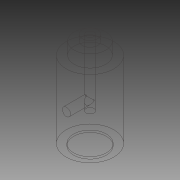
# Autodesk Inventor part: ToolHolderSlug Body
Saved by Autodesk Inventor 2012 SP1 (Build 160190100, 190)
## iProperties
Created: 2010-02-09
Part Number: ToolHolderSlug Body
Document SubType Name: Modeling
Designer: rconnaug
Density: 2.71 g/cm^3
Material: Aluminum-6061
Mass: 6.06549 g
Surface Area: 11.541 cm^2
Volume: 2.23819 cm^3
Author: rconnaug
Autodesk Inventor part; units mm, degrees
ref_plane "YZ Plane" through (0, 0, 0) normal (1, 0, 0) x (0, 1, 0)
ref_plane "XZ Plane" through (0, 0, 0) normal (0, 1, 0) x (-1, 0, 0)
sketch "Sketch1" plane through (0, 0, 0) normal (0, 0, 1) x (1, 0, 0)
  line L0 (0, -4.814) -> (0, 28.884) construction
  line L1 (0.9906, 24.07) -> (1.9304, 24.07)
  line L2 (1.9304, 24.07) -> (1.9304, 22.606)
  line L3 (1.9304, 22.606) -> (3.9497, 22.606)
  line L4 (3.9497, 22.606) -> (3.9497, 19.558)
  line L5 (3.9497, 19.558) -> (5.9246, 19.558)
  line L6 (5.9246, 19.558) -> (5.9246, 0.508)
  line L7 (0, 7.56) -> (0.9906, 7.56)
  line L8 (0.9906, 7.56) -> (0.9906, 24.07)
  line L9 (5.9246, 0.508) -> (4.075, 0.508)
  line L10 (4.075, 0.508) -> (4.075, 0)
  line L11 (4.075, 0) -> (0, 0)
  line L12 (0, 7.56) -> (0, 0)
  dimension "d0" = 5.9245
  dimension "d1" = 3.9497
  dimension "d2" = 0.9906
  dimension "d3" = 4.075
  dimension "d4" = 0.508
  dimension "d5" = 24.07
  dimension "d7" = 22.606
  dimension "d16" = 16.51
  dimension "d21" = 1.9304
  dimension "d40" = 19.05
  constraints: 24 end point, 5 parallel, 5 perpendicular, 1 collinear, 1 point on line
  measures "d0" distance between parallel lines of L0 L6
  measures "d1" distance between parallel lines of L0 L4
  measures "d2" distance between parallel lines of L0 L8
  measures "d3" distance between parallel lines of L0 L10
  measures "d4" distance between parallel lines of L9 L11
  measures "d5" distance between parallel lines of L11 L1
  measures "d7" distance between parallel lines of L11 L3
  measures "d16" distance between parallel lines of L1 L7
  measures "d21" distance between parallel lines of L0 L2
  measures "d40" distance of L5.end L6.end
revolve "Revolution1" add sketch "Sketch1" angle 360 about axis through (0, 7.56, 0) along (0, -1, 0)
ref_plane "Work Plane1" through (0, 10.033, 5.9246) normal (0, 0, 1) x (1, 0, 0)
sketch "Sketch7" plane through (0, 10.033, 5.9246) normal (0, 0, 1) x (1, 0, 0)
  line L0 (-0.9906, -2.473) -> (0.9906, -2.473) construction
  line L1 (0, -2.473) -> (0, 2.056) construction
  line L2 (-5.9246, -9.525) -> (5.9246, -9.525) construction
  point P0 (0, -10.033)
  point P1 (0, 0.254)
  dimension "d41" = 9.779
  constraints: 2 end point, 1 midpoint, 1 perpendicular, 1 point on line
  measures "d41" distance from line of point (0, 0.254) L2
hole "Hole2" at (0, 10.287, 5.9246) direction (0, 0, -1) diameter 2.032 depth 5.9182
body "Solid1"
